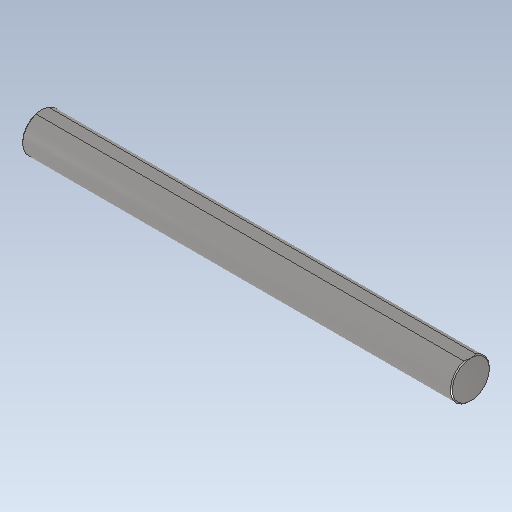
# Autodesk Inventor part: wał_półkola
Saved by Autodesk Inventor 2020 (Build 240168000, 168)
## iProperties
Created: 2020-08-21
Part Number: wał_półkola
Material: Stainless Steel
Document SubType Name: Modeling
Designer: Hesekiel
Density: 8 g/cm^3
Appearance: Semi-Polished
Mass: 549.124 g
Surface Area: 143.888 cm^2
Volume: 68.6405 cm^3
Author: Hesekiel
Autodesk Inventor part; units mm, degrees
ref_plane "XZ Plane" through (0, 0, 0) normal (0, 1, 0) x (-1, 0, 0)
ref_plane "XY Plane" through (0, 0, 0) normal (0, 0, 1) x (1, 0, 0)
sketch "Sketch1" plane through (0, 0, 0) normal (0, 1, 0) x (-1, 0, 0)
  circle A0 centre (0, 0) radius 10
  dimension "d0" = 20
  constraints: 1 centre point, 1 coincident
  measures "d0" diameter of A0
extrude "Extrusion1" add sketch "Sketch1" along normal blind 220
ref_plane "Work Plane1" through (10, 0, 0) normal (1, 0, 0) x (0, 1, 0)
sketch "Sketch2" plane through (10, 0, 0) normal (1, 0, 0) x (0, 1, 0)
  line L0 (220, -10) -> (220, 10) projected
  line L1 (0, -10) -> (0, 10) projected
  line L2 (0, 0) -> (132.5, 0)
  circle A0 centre (132.5, 0) radius 1.25
  circle A1 centre (132.5, 0) radius 0.5
  circle A2 centre (132.5, 0.0309) radius 2.5
  line L3 (0, -10) -> (0, 10) projected
  line L4 (132.5, -2.4691) -> (0, -2.4691)
  line L5 (0, -2.4691) -> (0, 2.5309)
  line L6 (0, 2.5309) -> (132.5, 2.5309)
  line L7 (132.5, 2.5309) -> (132.5, -2.4691)
  line L8 (220, -10) -> (220, 10) projected
  line L9 (132.5, -2.4691) -> (220, -2.4691)
  line L10 (220, -2.4691) -> (220, 2.5309)
  line L11 (220, 2.5309) -> (132.5, 2.5309)
  line L12 (132.5, 2.5309) -> (132.5, -2.4691)
  dimension "d21" = 5
  dimension "d3" = 132.5
  dimension "d4" = 2.5
  dimension "d5" = 1
  constraints: 18 end point, 4 parallel, 3 horizontal, 2 centre point, 2 coincident, 2 perpendicular, 2 point on line, 3 other
  measures "d3" distance of L2.start L2.end
  measures "d4" diameter of A0
  measures "d5" diameter of A1
extrude "Extrusion2" cut sketch "Sketch2" against normal blind 0.5
sketch "Sketch3" plane through (9.5, 0, 0) normal (1, 0, 0) x (0, 0, -1)
  line L0 (2.4691, 0) -> (-2.5309, 0) projected
  circle A0 centre (-0.0309, 132.5) radius 0.75
  circle A1 centre (-0.0309, 132.5) radius 1.25
  line L1 (2.4691, 220) -> (2.4691, 0) projected
  line L2 (-2.5309, 220) -> (2.4691, 220) projected
  line L3 (-2.5309, 0) -> (-2.5309, 220) projected
  point P0 (0, 0)
  dimension "d24" = 1.5
  dimension "d25" = 2.5
  constraints: 2 centre point, 1 coincident
  measures "d24" diameter of A0
  measures "d25" diameter of A1
extrude "Extrusion4" [suppressed]
chamfer "Chamfer5" [suppressed]
chamfer "Chamfer6" distance 0.5 angle 45 2 edges at (-9.9999, 220, -0.0319) (-9.9999, 0, -0.0319)
sketch "Sketch4" plane through (9.5, 0.3156, -2.4691) normal (0, 0, 1) x (1, 0, 0)
  spline S0 degree 2 poles (0.1904, 0.1843) (0.0943, 0.0912) (0, -0.0001) knots 0 0 0 1 1 1 weights 1 1.000046 1 projected
  line L0 (0.1904, 219.1844) -> (0.1904, 0.1844) projected
  spline S1 degree 4 poles (0, 219.3688) (0.0476, 219.3228) (0.0952, 219.2767) (0.1428, 219.2306) (0.1904, 219.1845) knots 0 0 0 0 0 1 1 1 1 1 projected
  line L1 (0, 219.3687) -> (0, 0) projected
  point P0 (-9.5, -0.3156)
  constraints: 2 other
extrude "Extrusion5" cut sketch "Sketch4" against normal blind 10
sketch "Sketch5" plane through (9.5, 0.3313, 2.5309) normal (0, 0, -1) x (-1, 0, 0)
  spline S0 degree 2 poles (0, -0.0001) (-0.0865, 0.0835) (-0.1744, 0.1686) knots 0 0 0 1 1 1 weights 1 1.000039 1 projected
  line L0 (0, 0) -> (0, 219.3373) projected
  spline S1 degree 2 poles (-0.1744, 219.1688) (-0.0865, 219.2539) (0, 219.3374) knots 0 0 0 1 1 1 weights 1 1.000039 1 projected
  line L1 (-0.1744, 0.1687) -> (-0.1744, 219.1687) projected
  point P0 (9.5, -0.3313)
  constraints: 2 other
extrude "Extrusion6" cut sketch "Sketch5" against normal blind 10
body "Solid1"
